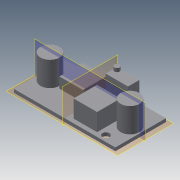
# Autodesk Inventor part: DC-DCconverter
Saved by Autodesk Inventor 2015 SP1 (Build 190203100, 203)
## iProperties
Created: 2015-02-22
Part Number: DC-DCconverter
Material: 一般
Document SubType Name: Modeling
Designer: Yamaura
Density: 1 g/cm^3
Appearance: 既定
Author: Yamaura
Autodesk Inventor part; units mm, degrees
sketch "スケッチ1" plane through (0, 0, 0) normal (0, 0, 1) x (1, 0, 0)
  line L0 (-21.5, 10.75) -> (21.5, 10.75)
  line L1 (21.5, 10.75) -> (21.5, -10.75)
  line L2 (21.5, -10.75) -> (-21.5, -10.75)
  line L3 (-21.5, -10.75) -> (-21.5, 10.75)
  line L4 (-21.5, -10.75) -> (21.5, 10.75)
  line L5 (-21.5, 10.75) -> (21.5, -10.75)
  point P0 (0, 0)
  dimension "d0" = 43
  dimension "d1" = 21.5
  constraints: 12 end point, 2 midpoint, 2 parallel, 1 horizontal, 1 perpendicular
  measures "d0" distance of L0.start L0.end
  measures "d1" distance of L0.end L1.end
extrude "押し出し1" add sketch "スケッチ1" along normal blind 1.4
sketch "スケッチ2" plane through (0, 0, 0) normal (0, 0, -1) x (-1, 0, 0)
  circle A0 centre (-15, -8.25) radius 1.5
  point P0 (0, 0)
  dimension "d4" = 3
  dimension "d5" = 15
  dimension "d6" = 8.25
  constraints: 1 centre point
  measures "d4" diameter of A0
  measures "d5" horizontal distance of A0.centre point (0, 0)
  measures "d6" vertical distance of A0.centre point (0, 0)
extrude "押し出し2" cut sketch "スケッチ2" against normal through all
sketch "スケッチ3" plane through (0, 0, 0) normal (0, 0, -1) x (-1, 0, 0)
  circle A0 centre (-17, 0) radius 4
  line L0 (-2, -9) -> (-12, -9)
  line L1 (-12, -9) -> (-12, 1)
  line L2 (-12, 1) -> (-2, 1)
  line L3 (-2, 1) -> (-2, -9)
  point P0 (0, 0)
  dimension "d12" = 8
  dimension "d13" = 17
  dimension "d16" = 10
  dimension "d17" = 10
  dimension "d18" = 2
  dimension "d23" = 1
  constraints: 8 end point, 2 parallel, 1 centre point, 1 horizontal, 1 horizontal alignment, 1 perpendicular
  measures "d12" diameter of A0
  measures "d13" distance of A0.centre point (0, 0)
  measures "d16" distance of L1.end L2.end
  measures "d17" distance of L0.end L1.end
  measures "d18" distance from line of L3 point (0, 0)
  measures "d23" distance from line of L2 point (0, 0)
extrude "押し出し3" add sketch "スケッチ3" against normal blind 11.8
pattern_circular "円形状パターン2" count 2 over 360 about axis through (0, 0, -10) along (0, 0, 1) of "押し出し3", "押し出し2"
sketch "スケッチ4" plane through (0, 0, 0) normal (0, 0, -1) x (-1, 0, 0)
  line L0 (-2.2, 4.45) -> (-11.7, 4.45)
  line L1 (-11.7, 4.45) -> (-11.7, 9.25)
  line L2 (-11.7, 9.25) -> (-2.2, 9.25)
  line L3 (-2.2, 9.25) -> (-2.2, 4.45)
  circle A0 centre (15, 8.25) radius 1.5 projected
  circle A1 centre (-15, -8.25) radius 1.5 projected
  line L4 (21.5, -10.75) -> (-21.5, -10.75) projected
  line L5 (21.5, 10.75) -> (21.5, -10.75) projected
  line L6 (-21.5, 10.75) -> (21.5, 10.75) projected
  line L7 (-21.5, -10.75) -> (-21.5, 10.75) projected
  point P0 (0, 0)
  dimension "d24" = 9.5
  dimension "d25" = 4.8
  dimension "d26" = 1.5
  dimension "d27" = 9.8
  constraints: 8 end point, 2 parallel, 1 horizontal, 1 perpendicular
  measures "d24" distance of L0.start L0.end
  measures "d25" distance of L2.end L0.start
  measures "d26" distance between parallel lines of L6 L2
  measures "d27" distance between parallel lines of L7 L1
extrude "押し出し4" add sketch "スケッチ4" against normal blind 11.3 contours L0 L1 L2 L3
sketch "スケッチ5" plane through (0, 0, 11.3) normal (0, 0, 1) x (1, 0, 0)
  line L0 (2.2, 4.45) -> (11.7, 4.45) projected
  line L1 (11.7, 4.45) -> (11.7, 9.25) projected
  line L2 (11.7, 9.25) -> (2.2, 9.25) projected
  line L3 (2.2, 9.25) -> (2.2, 4.45) projected
  circle A0 centre (3.3, 8.15) radius 1.1
  point P0 (0, 0)
  dimension "d30" = 2.2
  constraints: 2 tangent, 1 centre point
  measures "d30" diameter of A0
extrude "押し出し5" add sketch "スケッチ5" along normal blind 1.5 contours A0
move faces "移動1" translate (0, 0, -3) faces at (8.6667, -2.3333, 11.8)
move faces "移動2" translate (0, 0, -5.9) faces at (-5.3333, 5.6667, 11.8)
